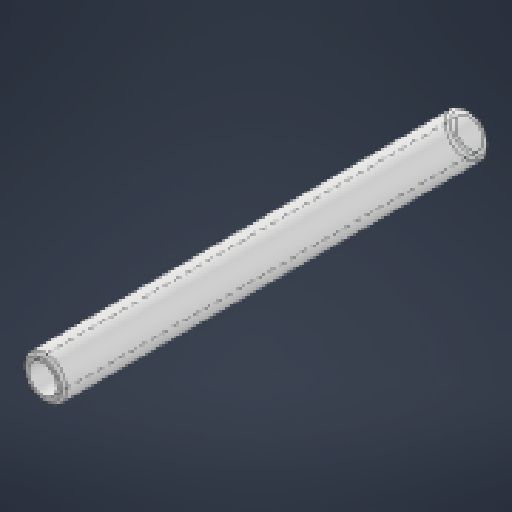
# Autodesk Inventor part: hollow linear shaft
Saved by Autodesk Inventor 2023 (Build 270158000, 158)
## iProperties
Created: 2025-09-04
Part Number: hollow linear shaft
Material: 일반
Document SubType Name: Modeling
Designer: k
Density: 1 g/cm^3
Appearance: 기본값
Author: k
Autodesk Inventor part; units mm, degrees
ref_plane "YZ Plane" through (0, 0, 0) normal (1, 0, 0) x (0, 1, 0)
ref_plane "XZ Plane" through (0, 0, 0) normal (0, 1, 0) x (-1, 0, 0)
ref_plane "XY Plane" through (0, 0, 0) normal (0, 0, 1) x (1, 0, 0)
sketch "스케치1" plane through (0, 0, 0) normal (0, 0, 1) x (1, 0, 0)
  circle A0 centre (-78.3854, 75.1255) radius 15
  circle A1 centre (-78.3854, 75.1255) radius 10
  point P0 (0, 0)
  dimension "d0" = 30
  dimension "d1" = 20
  constraints: 2 centre point, 1 coincident
  measures "d0" diameter of A0
  measures "d1" diameter of A1
extrude "돌출1" add sketch "스케치1" along normal blind 300
chamfer "모따기1" distance 2 angle 45 2 edges at (-93.3854, 75.1255, 300) (-93.3854, 75.1255, 0)
